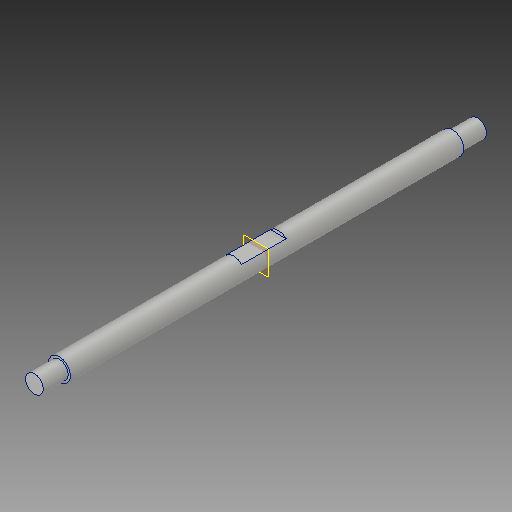
# Autodesk Inventor part: First stage shaft
Saved by Autodesk Inventor 2019.4 (Build 234330000, 330)
## iProperties
Created: 2020-01-19
Part Number: First stage shaft
Material: Aluminum 6061
Document SubType Name: Modeling
Designer: Mark
Mass: 40.0905 g
Surface Area: 62.6663 cm^2
Volume: 14.8483 cm^3
Density: 2.7 g/cm^3
Appearance: Aluminum - Flat
Author: Mark
Autodesk Inventor part; units mm, degrees
ref_plane "YZ Plane" through (0, 0, 0) normal (1, 0, 0) x (0, 1, 0)
ref_plane "XZ Plane" through (0, 0, 0) normal (0, 1, 0) x (-1, 0, 0)
ref_plane "XY Plane" through (0, 0, 0) normal (0, 0, 1) x (1, 0, 0)
sketch "Sketch1" plane through (0, 0, 0) normal (0, 0, 1) x (1, 0, 0)
  circle A0 centre (0, 0) radius 5
  dimension "d0" = 10
  constraints: 1 centre point, 1 coincident
  measures "d0" diameter of A0
extrude "Extrusion1" add sketch "Sketch1" along normal blind 199
sketch "Sketch2" plane through (0, 0, 199) normal (0, 0, 1) x (1, 0, 0)
  circle A0 centre (0, 0) radius 5
  circle A1 centre (0, 0) radius 4
  dimension "d3" = 10
  dimension "d4" = 8
  constraints: 2 centre point, 2 coincident
  measures "d3" diameter of A0
  measures "d4" diameter of A1
extrude "Extrusion2" cut sketch "Sketch2" against normal blind 11.2
sketch "Sketch3" plane through (0, 0, 0) normal (0, 0, -1) x (-1, 0, 0)
  circle A0 centre (0, 0) radius 5
  circle A1 centre (0, 0) radius 4
  dimension "d7" = 10
  dimension "d8" = 8
  constraints: 2 centre point, 2 coincident
  measures "d7" diameter of A0
  measures "d8" diameter of A1
extrude "Extrusion3" cut sketch "Sketch3" against normal blind 11.2
ref_plane "Work Plane1" through (0, 0, 99.5) normal (0, 0, 1) x (1, 0, 0)
sketch "Sketch4" plane through (0, 0, 99.5) normal (0, 0, 1) x (1, 0, 0)
  circle A0 centre (0, 0) radius 5
  line L0 (-5, 3.5) -> (5, 3.5)
  line L1 (5, 3.5) -> (5, 6.5)
  line L2 (5, 6.5) -> (-5, 6.5)
  line L3 (-5, 6.5) -> (-5, 3.5)
  line L4 (-5, 3.5) -> (5, 6.5) construction
  line L5 (5, 3.5) -> (-5, 6.5) construction
  point P0 (0, 5)
  dimension "d12" = 10
  dimension "d13" = 10
  dimension "d14" = 3
  constraints: 12 end point, 2 midpoint, 2 parallel, 1 coincident, 1 horizontal, 1 perpendicular, 1 vertical alignment, 2 other
  measures "d13" distance of L2.end L1.end
  measures "d14" distance of L1.end L0.end
extrude "Extrusion4" cut sketch "Sketch4" along normal mid plane 20 contours L0 A0 | A0 L0 L3 L2 L1 picked at (-0.189, 3.9893)
body "Solid1"
